Autodesk Fusion 360 part; units mm, degrees
note: some values were not read from the file. Set by a fixed rule: which face or edge a step refers to.
(part 2 of 5)
sketch "Sketch1 (5)" plane through (0, -26.65, 0) normal (0, -1, 0) x (1, 0, 0) in component "Servo_Mounting_Plate_1"
  line L0 (92.5, -27.97) -> (92.5, -18.97)
  line L1 (92.5, -18.97) -> (112.5, -18.97)
  line L2 (112.5, -18.97) -> (112.5, -27.97)
  line L3 (112.5, -27.97) -> (92.5, -27.97)
  circle A0 centre (11.5, -70.07) radius 1
  circle A1 centre (11.5, -4.1) radius 1
  circle A2 centre (11.5, -29.93) radius 1
  line L4 (92.5, -81.36) -> (92.5, -72.36)
  line L5 (92.5, -72.36) -> (112.5, -72.36)
  line L6 (112.5, -72.36) -> (112.5, -81.36)
  line L7 (112.5, -81.36) -> (92.5, -81.36)
  circle A3 centre (89.585, -23.47) radius 1
  circle A4 centre (115.415, -76.86) radius 1
  line L8 (16, -72.97) -> (16, -93)
  line L9 (16, -93) -> (7, -93)
  line L10 (7, -93) -> (7, -72.97)
  line L11 (7, -72.97) -> (16, -72.97)
  line L12 (16, -7) -> (16, -27.03)
  line L13 (16, -27.03) -> (7, -27.03)
  line L14 (7, -27.03) -> (7, -7)
  line L15 (7, -7) -> (16, -7)
  circle A5 centre (11.5, -95.9) radius 1
  circle A6 centre (89.585, -76.86) radius 1
  circle A7 centre (115.415, -23.47) radius 1
  line L16 (127.5, -73.5) -> (124.5, -73.5)
  line L17 (124.5, -73.5) -> (124.5, -68.5)
  line L18 (124.5, -68.5) -> (127.5, -68.5)
  line L19 (127.5, -68.5) -> (127.5, -73.5)
  line L20 (183.5, -73.5) -> (180.5, -73.5)
  line L21 (180.5, -73.5) -> (180.5, -68.5)
  line L22 (180.5, -68.5) -> (183.5, -68.5)
  line L23 (183.5, -68.5) -> (183.5, -73.5)
  line L24 (127.5, -31.5) -> (124.5, -31.5)
  line L25 (124.5, -31.5) -> (124.5, -26.5)
  line L26 (124.5, -26.5) -> (127.5, -26.5)
  line L27 (127.5, -26.5) -> (127.5, -31.5)
  line L28 (183.5, -31.5) -> (180.5, -31.5)
  line L29 (180.5, -31.5) -> (180.5, -26.5)
  line L30 (180.5, -26.5) -> (183.5, -26.5)
  line L31 (183.5, -26.5) -> (183.5, -31.5)
  arc A8 (157, -3) -> (154, 0) centre (154, -3) ccw
  line L32 (154, 0) -> (3, 0)
  arc A9 (3, 0) -> (0, -3) centre (3, -3) ccw
  line L33 (0, -3) -> (0, -97)
  arc A10 (0, -97) -> (3, -100) centre (3, -97) ccw
  line L34 (3, -100) -> (154, -100)
  arc A11 (154, -100) -> (157, -97) centre (154, -97) ccw
  line L35 (157, -97) -> (157, -94)
  arc A12 (160, -91) -> (157, -94) centre (160, -94) ccw
  line L36 (160, -91) -> (181.27, -91)
  arc A13 (181.27, -91) -> (184.27, -88) centre (181.27, -88) ccw
  line L37 (184.27, -88) -> (184.27, -12)
  arc A14 (184.27, -12) -> (181.27, -9) centre (181.27, -12) ccw
  line L38 (181.27, -9) -> (160, -9)
  arc A15 (157, -6) -> (160, -9) centre (160, -6) ccw
  line L39 (157, -6) -> (157, -3)
  line L40 (36.83, -3.81) -> (36.83, -13.97)
  line L41 (36.83, -13.97) -> (19.05, -13.97)
  line L42 (19.05, -13.97) -> (19.05, -3.81)
  line L43 (19.05, -3.81) -> (36.83, -3.81)
  line L44 (36.83, -96.52) -> (19.05, -96.52)
  line L45 (19.05, -96.52) -> (19.05, -86.36)
  line L46 (19.05, -86.36) -> (36.83, -86.36)
  line L47 (36.83, -86.36) -> (36.83, -96.52)
  line L48 (114.3, -3.81) -> (130.81, -3.81)
  line L49 (130.81, -3.81) -> (130.81, -13.97)
  line L50 (130.81, -13.97) -> (114.3, -13.97)
  line L51 (114.3, -13.97) -> (114.3, -3.81)
  line L52 (114.3, -96.52) -> (114.3, -86.36)
  line L53 (114.3, -86.36) -> (130.81, -86.36)
  line L54 (130.81, -86.36) -> (130.81, -96.52)
  line L55 (130.81, -96.52) -> (114.3, -96.52)
  circle A16 centre (115.415, -76.86) radius 1
  circle A17 centre (89.585, -76.86) radius 1
  line L56 (92.5, -76.86) -> (112.5, -76.86) construction
  line L57 (102.5, -72.36) -> (102.5, -81.36) construction
  line L58 (117.5, -86.25) -> (87.5, -86.25)
  line L59 (87.5, -86.25) -> (87.5, -67.47)
  line L60 (87.5, -67.47) -> (117.5, -67.47)
  line L61 (117.5, -67.47) -> (117.5, -86.25)
  line L62 (117.5, -86.25) -> (87.5, -67.47) construction
  line L63 (87.5, -86.25) -> (117.5, -67.47) construction
  line L64 (104.5, -72.36) -> (104.5, -81.36)
  line L65 (104.5, -72.36) -> (92.5, -72.36)
  line L66 (92.5, -72.36) -> (92.5, -81.36)
  line L67 (92.5, -81.36) -> (104.5, -81.36)
  point P0 (102.5, -76.86)
  dimension "d167" = 30
  dimension "d168" = 12
  constraint midpoint L4 L56.start
  constraint midpoint L6 L56.end
  constraint midpoint L5 L57.start
  constraint midpoint L7 L57.end
  constraint horizontal L58
  constraint perpendicular L58 L59
  constraint parallel L58 L60
  constraint parallel L59 L61
  constraint coincident L62 P0
  constraint coincident L63 P0
  constraint midpoint L57 P0
  constraint coincident L5 L64.start
  constraint coincident L7 L64.end
  constraint perpendicular L7 L64
  constraint coincident L4.end L5.start
  constraint coincident L4.start L7.end
  measures "d167" distance of L59.end L60.end
  measures "d168" distance of L4 L64
extrude "Extrude1''''''" add sketch "Sketch1 (5)" along normal blind 5.45 separate body contours L5 L6 L7 L64 | A4 A16 | A6 A17 | L58 L59 L60 L61 makes body 11 in component "Servo_Mounting_Plate_1"
sketch "Sketch2 (5)" plane through (0, -32.1, 0) normal (0, -1, 0) x (1, 0, 0) in component "Servo_Mounting_Plate_1"
  line L0 (92.5, -72.36) -> (104.5, -72.36)
  line L1 (104.5, -72.36) -> (104.5, -81.36)
  line L2 (104.5, -81.36) -> (92.5, -81.36)
  line L3 (92.5, -81.36) -> (92.5, -72.36)
  line L4 (117.5, -67.47) -> (87.5, -67.47)
  line L5 (87.5, -67.47) -> (87.5, -86.25)
  line L6 (87.5, -86.25) -> (117.5, -86.25)
  line L7 (117.5, -86.25) -> (117.5, -67.47)
  line L8 (92.5, -76.86) -> (96.3, -76.86) construction
  circle A0 centre (96.3, -76.86) radius 8.2
  circle A1 centre (96.3, -76.86) radius 10.2
  dimension "d171" = 3.8
  dimension "d172" = 2
  constraint midpoint L3 L8.start
  constraint perpendicular L3 L8
  constraint coincident L8.end A0.centre
  constraint tangent L1 A0
  measures "d171" distance of L8.start L8.end
extrude "Extrude2''''" cut sketch "Sketch2 (5)" against normal blind 2 contours L4 L5 L6 A1 bodies 11 in component "Servo_Mounting_Plate_1"
sketch "Sketch3 (3)" plane through (0, -26.65, 0) normal (0, 1, 0) x (-1, 0, 0) in component "Servo_Mounting_Plate_1"
  line L0 (-104.5, -72.36) -> (-92.5, -72.36)
  line L1 (-92.5, -72.36) -> (-92.5, -81.36)
  line L2 (-92.5, -81.36) -> (-104.5, -81.36)
  line L3 (-104.5, -81.36) -> (-104.5, -72.36)
  line L4 (-87.5, -67.47) -> (-117.5, -67.47)
  line L5 (-117.5, -67.47) -> (-117.5, -86.25)
  line L6 (-117.5, -86.25) -> (-87.5, -86.25)
  line L7 (-87.5, -86.25) -> (-87.5, -67.47)
  circle A0 centre (-90, -84) radius 0.95
  circle A1 centre (-90, -69.72) radius 0.95
  circle A2 centre (-114, -84) radius 0.95
  circle A3 centre (-114, -69.72) radius 0.95
  dimension "d175" = 2.25
  dimension "d176" = 2.25
  dimension "d177" = 2.25
  dimension "d178" = 2.25
  dimension "d314" = 1.9
  dimension "d315" = 24
  dimension "d316" = 1.9
  dimension "d317" = 1.9
  dimension "d318" = 1.9
  measures "d175" distance of L6 A0.centre
  measures "d176" distance of L4 A1.centre
  measures "d177" distance of L6 A2.centre
  measures "d178" distance of L4 A3.centre
  measures "d314" diameter of A0
  measures "d315" distance of A0.centre A2.centre
  measures "d316" diameter of A2
  measures "d317" diameter of A3
  measures "d318" diameter of A1
extrude "Extrude3''" add sketch "Sketch3 (3)" along normal blind 1 contours A0 | A1 | A2 | A3 bodies 11 in component "Servo_Mounting_Plate_1"
sketch "Sketch18" plane through (0, -26.65, 0) normal (0, -1, 0) x (1, 0, 0) in component "Chassis"
  line L0 (92.5, -27.97) -> (92.5, -18.97)
  line L1 (92.5, -18.97) -> (112.5, -18.97)
  line L2 (112.5, -18.97) -> (112.5, -27.97)
  line L3 (112.5, -27.97) -> (92.5, -27.97)
  circle A0 centre (11.5, -70.07) radius 1
  circle A1 centre (11.5, -4.1) radius 1
  circle A2 centre (11.5, -29.93) radius 1
  line L4 (92.5, -81.36) -> (92.5, -72.36)
  line L5 (92.5, -72.36) -> (112.5, -72.36)
  line L6 (112.5, -72.36) -> (112.5, -81.36)
  line L7 (112.5, -81.36) -> (92.5, -81.36)
  circle A3 centre (89.585, -23.47) radius 1
  circle A4 centre (115.415, -76.86) radius 1
  line L8 (16, -72.97) -> (16, -93)
  line L9 (16, -93) -> (7, -93)
  line L10 (7, -93) -> (7, -72.97)
  line L11 (7, -72.97) -> (16, -72.97)
  line L12 (16, -7) -> (16, -27.03)
  line L13 (16, -27.03) -> (7, -27.03)
  line L14 (7, -27.03) -> (7, -7)
  line L15 (7, -7) -> (16, -7)
  circle A5 centre (11.5, -95.9) radius 1
  circle A6 centre (89.585, -76.86) radius 1
  circle A7 centre (115.415, -23.47) radius 1
  line L16 (127.5, -73.5) -> (124.5, -73.5)
  line L17 (124.5, -73.5) -> (124.5, -68.5)
  line L18 (124.5, -68.5) -> (127.5, -68.5)
  line L19 (127.5, -68.5) -> (127.5, -73.5)
  line L20 (183.5, -73.5) -> (180.5, -73.5)
  line L21 (180.5, -73.5) -> (180.5, -68.5)
  line L22 (180.5, -68.5) -> (183.5, -68.5)
  line L23 (183.5, -68.5) -> (183.5, -73.5)
  line L24 (127.5, -31.5) -> (124.5, -31.5)
  line L25 (124.5, -31.5) -> (124.5, -26.5)
  line L26 (124.5, -26.5) -> (127.5, -26.5)
  line L27 (127.5, -26.5) -> (127.5, -31.5)
  line L28 (183.5, -31.5) -> (180.5, -31.5)
  line L29 (180.5, -31.5) -> (180.5, -26.5)
  line L30 (180.5, -26.5) -> (183.5, -26.5)
  line L31 (183.5, -26.5) -> (183.5, -31.5)
  arc A8 (157, -3) -> (154, 0) centre (154, -3) ccw
  line L32 (154, 0) -> (3, 0)
  arc A9 (3, 0) -> (0, -3) centre (3, -3) ccw
  line L33 (0, -3) -> (0, -97)
  arc A10 (0, -97) -> (3, -100) centre (3, -97) ccw
  line L34 (3, -100) -> (154, -100)
  arc A11 (154, -100) -> (157, -97) centre (154, -97) ccw
  line L35 (157, -97) -> (157, -94)
  arc A12 (160, -91) -> (157, -94) centre (160, -94) ccw
  line L36 (160, -91) -> (181.27, -91)
  arc A13 (181.27, -91) -> (184.27, -88) centre (181.27, -88) ccw
  line L37 (184.27, -88) -> (184.27, -12)
  arc A14 (184.27, -12) -> (181.27, -9) centre (181.27, -12) ccw
  line L38 (181.27, -9) -> (160, -9)
  arc A15 (157, -6) -> (160, -9) centre (160, -6) ccw
  line L39 (157, -6) -> (157, -3)
  line L40 (36.83, -3.81) -> (36.83, -13.97)
  line L41 (36.83, -13.97) -> (19.05, -13.97)
  line L42 (19.05, -13.97) -> (19.05, -3.81)
  line L43 (19.05, -3.81) -> (36.83, -3.81)
  line L44 (36.83, -96.52) -> (19.05, -96.52)
  line L45 (19.05, -96.52) -> (19.05, -86.36)
  line L46 (19.05, -86.36) -> (36.83, -86.36)
  line L47 (36.83, -86.36) -> (36.83, -96.52)
  line L48 (114.3, -3.81) -> (130.81, -3.81)
  line L49 (130.81, -3.81) -> (130.81, -13.97)
  line L50 (130.81, -13.97) -> (114.3, -13.97)
  line L51 (114.3, -13.97) -> (114.3, -3.81)
  line L52 (114.3, -96.52) -> (114.3, -86.36)
  line L53 (114.3, -86.36) -> (130.81, -86.36)
  line L54 (130.81, -86.36) -> (130.81, -96.52)
  line L55 (130.81, -96.52) -> (114.3, -96.52)
  circle A16 centre (90, -69.72) radius 1.0625
  circle A17 centre (90, -84) radius 1.0625
  circle A18 centre (114, -69.72) radius 1.0625
  circle A19 centre (114, -84) radius 1.0625
  line L56 (184.27, -50) -> (65, -50) construction
  circle A20 centre (90, -30.28) radius 1.0625
  circle A21 centre (114, -30.28) radius 1.0625
  circle A22 centre (114, -16) radius 1.0625
  circle A23 centre (90, -16) radius 1.0625
  point P0 (90, -69.72)
  point P1 (90, -84)
  point P2 (114, -84)
  point P3 (114, -69.72)
  dimension "d181" = 2.125
  dimension "d182" = 2.125
  dimension "d183" = 2.125
  dimension "d184" = 2.125
  constraint coincident P0 A16.centre
  constraint coincident P1 A17.centre
  constraint coincident P3 A18.centre
  constraint coincident P2 A19.centre
  constraint midpoint L37 L56.start
  constraint perpendicular L37 L56
  constraint symmetric A16 L56 A20
  constraint symmetric A17 L56 A23
  constraint symmetric A18 L56 A21
  constraint symmetric A19 L56 A22
  measures "d181" diameter of A16
  measures "d182" diameter of A17
  measures "d183" diameter of A18
  measures "d184" diameter of A19
extrude "Extrude17" cut sketch "Sketch18" against normal blind 1 contours A16 | A17 | A18 | A19 bodies 4 in component "Chassis"
extrude "Extrude18" cut sketch "Sketch18" against normal blind 1 contours A20 | A21 | A22 | A23 bodies 4 in component "Chassis"
sketch "Sketch1 (6)" plane through (0, -30.1, 0) normal (0, -1, 0) x (1, 0, 0) in component "Back_Wheel_L"
  arc A0 (103.1549, -72.36) -> (103.1549, -81.36) centre (96.3, -76.86) ccw
  line L0 (103.1549, -72.36) -> (104.5, -72.36)
  line L1 (104.5, -72.36) -> (104.5, -81.36)
  line L2 (104.5, -81.36) -> (103.1549, -81.36)
  arc A1 (100.2833, -86.25) -> (100.2833, -67.47) centre (96.3, -76.86) ccw
  line L3 (100.2833, -67.47) -> (92.3167, -67.47)
  arc A2 (92.3167, -67.47) -> (87.5, -71.7025) centre (96.3, -76.86) ccw
  line L4 (87.5, -71.7025) -> (87.5, -82.0175)
  arc A3 (87.5, -82.0175) -> (92.3167, -86.25) centre (96.3, -76.86) ccw
  line L5 (92.3167, -86.25) -> (100.2833, -86.25)
  circle A4 centre (96.3, -76.86) radius 10
  circle A5 centre (96.3, -76.86) radius 8.75
  dimension "d189" = 20
  dimension "d190" = -1.25
  constraint concentric A0 A4
  measures "d189" diameter of A4
extrude "Extrude1'''''''" add sketch "Sketch1 (6)" along normal blind 5.18 separate body contours L0 L1 A5 | L1 L2 A5 | L5 A4 | L3 L4 L5 A4 | L3 A4 | L4 A4 makes body 12 in component "Back_Wheel_L"
sketch "Sketch2 (6)" plane through (0, -35.28, 0) normal (0, -1, 0) x (1, 0, 0) in component "Back_Wheel_L"
  circle A0 centre (96.3, -76.86) radius 8.75
  circle A1 centre (96.3, -76.86) radius 10
  circle A2 centre (96.3, -76.86) radius 12
  dimension "d193" = 24
  constraint concentric A0 A2
  measures "d193" diameter of A2
extrude "Extrude2'''''" add sketch "Sketch2 (6)" against normal blind 3.15 contours A2 bodies 12 in component "Back_Wheel_L"
sketch "Sketch3 (4)" plane through (0, -35.28, 0) normal (0, -1, 0) x (1, 0, 0) in component "Back_Wheel_L"
  circle A0 centre (96.3, -76.86) radius 12
  circle A1 centre (96.3, -76.86) radius 8.75
  circle A2 centre (96.3, -76.86) radius 12
  constraint concentric A0 A2
extrude "Extrude3'''" add sketch "Sketch3 (4)" along normal blind 1 contours A0 A2 | A1 bodies 12 in component "Back_Wheel_L"
sketch "Sketch4 (3)" plane through (0, -36.28, 0) normal (0, -1, 0) x (1, 0, 0) in component "Back_Wheel_L"
  circle A0 centre (96.3, -76.86) radius 12
  circle A1 centre (96.3, -76.86) radius 8.75
  circle A2 centre (96.3, -76.86) radius 12
  constraint concentric A1 A2
extrude "Extrude4''" add sketch "Sketch4 (3)" along normal blind 10 bodies 12 in component "Back_Wheel_L"
sketch "Sketch5 (3)" plane through (0, -46.28, 0) normal (0, -1, 0) x (1, 0, 0) in component "Back_Wheel_L"
  circle A0 centre (96.3, -76.86) radius 8.75
  circle A1 centre (96.3, -76.86) radius 12
  line L0 (106, -76.86) -> (106, -69.7953)
  line L1 (106, -76.86) -> (106, -83.9247)
  line L2 (106, -83.9247) -> (111, -83.9247)
  line L3 (111, -83.9247) -> (111, -69.7953)
  line L4 (111, -69.7953) -> (106, -69.7953)
  line L5 (106, -69.7953) -> (106, -83.9247)
  dimension "d200" = 5
  constraint coincident A1 L0.end
  constraint coincident A1 L1.end
  constraint horizontal L2
  constraint vertical L3
  constraint horizontal L4
  constraint vertical L5
  measures "d200" distance of L1.end L2.end
extrude "Extrude5''" add sketch "Sketch5 (3)" against normal blind 10 contours A1 L2 L3 L4 bodies 12 in component "Back_Wheel_L"
sketch "Sketch6 (2)" plane through (0, 0, -83.9247) normal (0, 0, -1) x (-1, 0, 0) in component "Back_Wheel_L"
  line L0 (-111, -46.28) -> (-106, -46.28)
  line L1 (-106, -46.28) -> (-106, -36.28)
  line L2 (-106, -36.28) -> (-111, -36.28)
  line L3 (-111, -36.28) -> (-111, -46.28)
  line L4 (-111, -36.28) -> (-135.7487, -61.0287)
  line L5 (-111, -36.28) -> (-76, -36.28) construction
  line L6 (-135.7487, -61.0287) -> (-111, -46.28) construction
  line L7 (-135.7487, -61.0287) -> (-135.7487, -76.0287)
  line L8 (-135.7487, -76.0287) -> (-120.7487, -76.0287)
  line L9 (-120.7487, -76.0287) -> (-120.7487, -61.0287)
  line L10 (-111, -46.28) -> (-120.7487, -61.0287)
  dimension "d203" = 135
  dimension "d204" = 35
  dimension "d205" = 15
  dimension "d206" = 15
  dimension "d207" = 15
  constraint horizontal L5
  constraint coincident L2.end L3.start
  constraint coincident L0.start L3.end
  constraint vertical L7
  constraint perpendicular L7 L8
  constraint perpendicular L8 L9
  measures "d203" angle of L4 L5
  measures "d204" distance of L2.end L4.end
  measures "d205" distance of L4.end L7.end
  measures "d206" distance of L7.end L8.end
  measures "d207" distance of L8.end L9.end
extrude "Extrude6''" add sketch "Sketch6 (2)" against normal blind 14.129 contours L3 L4 L7 L8 L9 L10 bodies 12 in component "Back_Wheel_L"
sketch "Sketch1 (7)" plane through (0, -30.1, 0) normal (0, -1, 0) x (1, 0, 0) in component "Back_Wheel_R"
  arc A0 (103.1549, -72.36) -> (103.1549, -81.36) centre (96.3, -76.86) ccw
  line L0 (103.1549, -72.36) -> (104.5, -72.36)
  line L1 (104.5, -72.36) -> (104.5, -81.36)
  line L2 (104.5, -81.36) -> (103.1549, -81.36)
  arc A1 (100.2833, -86.25) -> (100.2833, -67.47) centre (96.3, -76.86) ccw
  line L3 (100.2833, -67.47) -> (92.3167, -67.47)
  arc A2 (92.3167, -67.47) -> (87.5, -71.7025) centre (96.3, -76.86) ccw
  line L4 (87.5, -71.7025) -> (87.5, -82.0175)
  arc A3 (87.5, -82.0175) -> (92.3167, -86.25) centre (96.3, -76.86) ccw
  line L5 (92.3167, -86.25) -> (100.2833, -86.25)
  circle A4 centre (96.3, -76.86) radius 10
  circle A5 centre (96.3, -76.86) radius 8.75
  dimension "d189_1" = 20
  dimension "d190_1" = -1.25
  constraint concentric A0 A4
  measures "d189_1" diameter of A4
extrude "Extrude1''''''''" add sketch "Sketch1 (7)" along normal blind 5.18 separate body contours L0 L1 A5 | L1 L2 A5 | L5 A4 | L3 L4 L5 A4 | L3 A4 | L4 A4 makes body 13 in component "Back_Wheel_R"
sketch "Sketch2 (7)" plane through (0, -35.28, 0) normal (0, -1, 0) x (1, 0, 0) in component "Back_Wheel_R"
  circle A0 centre (96.3, -76.86) radius 8.75
  circle A1 centre (96.3, -76.86) radius 10
  circle A2 centre (96.3, -76.86) radius 12
  dimension "d193_1" = 24
  constraint concentric A0 A2
  measures "d193_1" diameter of A2
extrude "Extrude2''''''" add sketch "Sketch2 (7)" against normal blind 3.15 contours A2 bodies 13 in component "Back_Wheel_R"
sketch "Sketch3 (5)" plane through (0, -35.28, 0) normal (0, -1, 0) x (1, 0, 0) in component "Back_Wheel_R"
  circle A0 centre (96.3, -76.86) radius 12
  circle A1 centre (96.3, -76.86) radius 8.75
  circle A2 centre (96.3, -76.86) radius 12
  constraint concentric A0 A2
extrude "Extrude3''''" add sketch "Sketch3 (5)" along normal blind 1 contours A0 A2 | A1 bodies 13 in component "Back_Wheel_R"
sketch "Sketch4 (4)" plane through (0, -36.28, 0) normal (0, -1, 0) x (1, 0, 0) in component "Back_Wheel_R"
  circle A0 centre (96.3, -76.86) radius 12
  circle A1 centre (96.3, -76.86) radius 8.75
  circle A2 centre (96.3, -76.86) radius 12
  constraint concentric A1 A2
extrude "Extrude4'''" add sketch "Sketch4 (4)" along normal blind 10 bodies 13 in component "Back_Wheel_R"
sketch "Sketch5 (4)" plane through (0, -46.28, 0) normal (0, -1, 0) x (1, 0, 0) in component "Back_Wheel_R"
  circle A0 centre (96.3, -76.86) radius 8.75
  circle A1 centre (96.3, -76.86) radius 12
  line L0 (106, -76.86) -> (106, -69.7953)
  line L1 (106, -76.86) -> (106, -83.9247)
  line L2 (106, -83.9247) -> (111, -83.9247)
  line L3 (111, -83.9247) -> (111, -69.7953)
  line L4 (111, -69.7953) -> (106, -69.7953)
  line L5 (106, -69.7953) -> (106, -83.9247)
  dimension "d200_1" = 5
  constraint coincident A1 L0.end
  constraint coincident A1 L1.end
  constraint horizontal L2
  constraint vertical L3
  constraint horizontal L4
  constraint vertical L5
  measures "d200_1" distance of L1.end L2.end
extrude "Extrude5'''" add sketch "Sketch5 (4)" against normal blind 10 contours A1 L2 L3 L4 bodies 13 in component "Back_Wheel_R"
sketch "Sketch6 (3)" plane through (0, 0, -83.9247) normal (0, 0, -1) x (-1, 0, 0) in component "Back_Wheel_R"
  line L0 (-111, -46.28) -> (-106, -46.28)
  line L1 (-106, -46.28) -> (-106, -36.28)
  line L2 (-106, -36.28) -> (-111, -36.28)
  line L3 (-111, -36.28) -> (-111, -46.28)
  line L4 (-111, -36.28) -> (-76, -36.28) construction
  line L5 (-135.7487, -61.0287) -> (-111, -46.28) construction
  line L6 (-135.7487, -61.0287) -> (-135.7487, -76.0287)
  line L7 (-135.7487, -76.0287) -> (-120.7487, -76.0287)
  line L8 (-120.7487, -76.0287) -> (-120.7487, -61.0287)
  line L9 (-120.7487, -61.0287) -> (-111, -46.28)
  line L10 (-111, -36.28) -> (-135.7487, -61.0287)
  dimension "d205_1" = 15
  dimension "d206_1" = 15
  dimension "d207_1" = 15
  constraint horizontal L4
  constraint coincident L2.end L3.start
  constraint coincident L0.start L3.end
  constraint vertical L6
  constraint perpendicular L6 L7
  constraint perpendicular L7 L8
  measures "d205_1" distance of L5.start L6.end
  measures "d206_1" distance of L6.end L7.end
  measures "d207_1" distance of L7.end L8.end
extrude "Extrude6'''" add sketch "Sketch6 (3)" against normal blind 14.129 contours L3 L6 L7 L8 L9 L10 bodies 13 in component "Back_Wheel_R"
sketch "Sketch2 (8)" plane through (0, -26.65, 0) normal (0, -1, 0) x (1, 0, 0) in component "Front_L_Servo_Mounting_Plate"
  circle A0 centre (90, -16) radius 1.0625
  circle A1 centre (114, -16) radius 1.0625
  circle A2 centre (90, -30.28) radius 1.0625
  circle A3 centre (114, -30.28) radius 1.0625
  circle A4 centre (114, -69.72) radius 1.0625
  circle A5 centre (90, -84) radius 1.0625
  circle A6 centre (90, -69.72) radius 1.0625
  circle A7 centre (114, -84) radius 1.0625
  line L0 (92.5, -27.97) -> (92.5, -18.97)
  line L1 (92.5, -18.97) -> (112.5, -18.97)
  line L2 (112.5, -18.97) -> (112.5, -27.97)
  line L3 (112.5, -27.97) -> (92.5, -27.97)
  circle A8 centre (11.5, -70.07) radius 1
  circle A9 centre (11.5, -4.1) radius 1
  circle A10 centre (11.5, -29.93) radius 1
  line L4 (92.5, -81.36) -> (92.5, -72.36)
  line L5 (92.5, -72.36) -> (112.5, -72.36)
  line L6 (112.5, -72.36) -> (112.5, -81.36)
  line L7 (112.5, -81.36) -> (92.5, -81.36)
  circle A11 centre (89.585, -23.47) radius 1
  circle A12 centre (115.415, -76.86) radius 1
  line L8 (16, -72.97) -> (16, -93)
  line L9 (16, -93) -> (7, -93)
  line L10 (7, -93) -> (7, -72.97)
  line L11 (7, -72.97) -> (16, -72.97)
  line L12 (16, -7) -> (16, -27.03)
  line L13 (16, -27.03) -> (7, -27.03)
  line L14 (7, -27.03) -> (7, -7)
  line L15 (7, -7) -> (16, -7)
  circle A13 centre (11.5, -95.9) radius 1
  circle A14 centre (89.585, -76.86) radius 1
  circle A15 centre (115.415, -23.47) radius 1
  line L16 (127.5, -73.5) -> (124.5, -73.5)
  line L17 (124.5, -73.5) -> (124.5, -68.5)
  line L18 (124.5, -68.5) -> (127.5, -68.5)
  line L19 (127.5, -68.5) -> (127.5, -73.5)
  line L20 (183.5, -73.5) -> (180.5, -73.5)
  line L21 (180.5, -73.5) -> (180.5, -68.5)
  line L22 (180.5, -68.5) -> (183.5, -68.5)
  line L23 (183.5, -68.5) -> (183.5, -73.5)
  line L24 (127.5, -31.5) -> (124.5, -31.5)
  line L25 (124.5, -31.5) -> (124.5, -26.5)
  line L26 (124.5, -26.5) -> (127.5, -26.5)
  line L27 (127.5, -26.5) -> (127.5, -31.5)
  line L28 (183.5, -31.5) -> (180.5, -31.5)
  line L29 (180.5, -31.5) -> (180.5, -26.5)
  line L30 (180.5, -26.5) -> (183.5, -26.5)
  line L31 (183.5, -26.5) -> (183.5, -31.5)
  arc A16 (157, -3) -> (154, 0) centre (154, -3) ccw
  line L32 (154, 0) -> (3, 0)
  arc A17 (3, 0) -> (0, -3) centre (3, -3) ccw
  line L33 (0, -3) -> (0, -97)
  arc A18 (0, -97) -> (3, -100) centre (3, -97) ccw
  line L34 (3, -100) -> (154, -100)
  arc A19 (154, -100) -> (157, -97) centre (154, -97) ccw
  line L35 (157, -97) -> (157, -94)
  arc A20 (160, -91) -> (157, -94) centre (160, -94) ccw
  line L36 (160, -91) -> (181.27, -91)
  arc A21 (181.27, -91) -> (184.27, -88) centre (181.27, -88) ccw
  line L37 (184.27, -88) -> (184.27, -12)
  arc A22 (184.27, -12) -> (181.27, -9) centre (181.27, -12) ccw
  line L38 (181.27, -9) -> (160, -9)
  arc A23 (157, -6) -> (160, -9) centre (160, -6) ccw
  line L39 (157, -6) -> (157, -3)
  line L40 (36.83, -3.81) -> (36.83, -13.97)
  line L41 (36.83, -13.97) -> (19.05, -13.97)
  line L42 (19.05, -13.97) -> (19.05, -3.81)
  line L43 (19.05, -3.81) -> (36.83, -3.81)
  line L44 (36.83, -96.52) -> (19.05, -96.52)
  line L45 (19.05, -96.52) -> (19.05, -86.36)
  line L46 (19.05, -86.36) -> (36.83, -86.36)
  line L47 (36.83, -86.36) -> (36.83, -96.52)
  line L48 (114.3, -3.81) -> (130.81, -3.81)
  line L49 (130.81, -3.81) -> (130.81, -13.97)
  line L50 (130.81, -13.97) -> (114.3, -13.97)
  line L51 (114.3, -13.97) -> (114.3, -3.81)
  line L52 (114.3, -96.52) -> (114.3, -86.36)
  line L53 (114.3, -86.36) -> (130.81, -86.36)
  line L54 (130.81, -86.36) -> (130.81, -96.52)
  line L55 (130.81, -96.52) -> (114.3, -96.52)
  line L56 (19.05, -86.36) -> (19.05, -100)
  line L57 (19.05, -100) -> (3, -100)
  line L58 (0, -97) -> (0, -68.36)
  line L59 (0, -68.36) -> (25, -68.36)
  line L60 (25, -68.36) -> (25, -86.36)
  line L61 (19.05, -86.36) -> (25, -86.36)
  arc A24 (0, -97) -> (3, -100) centre (3, -97) ccw
  line L62 (7, -72.97) -> (7, -84.97) construction
  line L63 (7, -84.97) -> (16, -84.97)
  dimension "d237" = 25
  dimension "d238" = 18
  dimension "d239" = 3
  dimension "d240" = 12
  constraint coincident L45.end L46.start
  constraint coincident L34 L56.end
  constraint perpendicular L34 L56
  constraint coincident A18.end L34.start
  constraint coincident L33.end A18.start
  constraint coincident L33 L58.end
  constraint perpendicular L34 L58
  constraint perpendicular L58 L59
  constraint coincident L46 L60.end
  constraint perpendicular L46 L60
  constraint coincident L10.end L11.start
  constraint perpendicular L11 L62
  constraint coincident L8 L63.end
  constraint perpendicular L8 L63
  measures "d237" distance of L58.end L59.end
  measures "d238" distance of L59.end L60.end
  measures "d239" radius of A24
  measures "d240" distance of L10.end L62.end
extrude "Extrude1'''''''''" add sketch "Sketch2 (8)" along normal blind 5.45 separate body contours A8 | L8 L9 L10 L63 | A13 | L33 A18 L34 L45 L46 L56 L57 L58 L59 L60 L61 A24 makes body 14 in component "Front_L_Servo_Mounting_Plate"
sketch "Sketch1 (8)" plane through (0, -32.1, 0) normal (0, -1, 0) x (1, 0, 0) in component "Front_L_Servo_Mounting_Plate"
  line L0 (7, -84.97) -> (7, -72.97)
  line L1 (7, -72.97) -> (16, -72.97)
  line L2 (16, -72.97) -> (16, -84.97)
  line L3 (16, -84.97) -> (7, -84.97)
  line L4 (0, -68.36) -> (0, -97)
  arc A0 (0, -97) -> (3, -100) centre (3, -97) ccw
  line L5 (3, -100) -> (19.05, -100)
  line L6 (19.05, -100) -> (19.05, -86.36)
  line L7 (19.05, -86.36) -> (25, -86.36)
  line L8 (25, -86.36) -> (25, -68.36)
  line L9 (25, -68.36) -> (0, -68.36)
  line L10 (11.5, -72.97) -> (11.5, -76.77) construction
  circle A1 centre (11.5, -76.77) radius 8.2
  circle A2 centre (11.5, -76.77) radius 10.2
  dimension "d243" = 3.8
  dimension "d244" = 2
  constraint midpoint L1 L10.start
  constraint perpendicular L1 L10
  constraint coincident L10.end A1.centre
  constraint tangent L3 A1
  measures "d243" distance of L10.start L10.end
extrude "Extrude2'''''''" cut sketch "Sketch1 (8)" against normal blind 2 contours L9 A2 picked at (13.8393, -85.5315) bodies 14 in component "Front_L_Servo_Mounting_Plate"
sketch "Sketch2 (9)" plane through (0, -26.65, 0) normal (0, 1, 0) x (-1, 0, 0) in component "Front_L_Servo_Mounting_Plate"
  line L0 (-7, -72.97) -> (-7, -84.97)
  line L1 (-7, -84.97) -> (-16, -84.97)
  line L2 (-16, -84.97) -> (-16, -72.97)
  line L3 (-16, -72.97) -> (-7, -72.97)
  line L4 (0, -97) -> (0, -68.36)
  line L5 (0, -68.36) -> (-25, -68.36)
  line L6 (-25, -68.36) -> (-25, -86.36)
  line L7 (-25, -86.36) -> (-19.05, -86.36)
  line L8 (-19.05, -86.36) -> (-19.05, -100)
  line L9 (-19.05, -100) -> (-3, -100)
  arc A0 (-3, -100) -> (0, -97) centre (-3, -97) ccw
  circle A1 centre (-3, -97) radius 0.95
  circle A2 centre (-22, -71) radius 0.95
  circle A3 centre (-3, -71) radius 0.95
  dimension "d247" = 1.9
  dimension "d249" = 1.9
  dimension "d250" = 1.9
  constraint concentric A0 A1
  measures "d247" diameter of A1
  measures "d249" diameter of A2
  measures "d250" diameter of A3
extrude "Extrude3'''''" add sketch "Sketch2 (9)" along normal blind 1 contours A1 | A2 | A3 bodies 14 in component "Front_L_Servo_Mounting_Plate"
sketch "Sketch19" plane through (0, -26.65, 0) normal (0, -1, 0) x (1, 0, 0) in component "Chassis"
  circle A0 centre (90, -16) radius 1.0625
  circle A1 centre (114, -16) radius 1.0625
  circle A2 centre (90, -30.28) radius 1.0625
  circle A3 centre (114, -30.28) radius 1.0625
  circle A4 centre (114, -69.72) radius 1.0625
  circle A5 centre (90, -84) radius 1.0625
  circle A6 centre (90, -69.72) radius 1.0625
  circle A7 centre (114, -84) radius 1.0625
  line L0 (92.5, -27.97) -> (92.5, -18.97)
  line L1 (92.5, -18.97) -> (112.5, -18.97)
  line L2 (112.5, -18.97) -> (112.5, -27.97)
  line L3 (112.5, -27.97) -> (92.5, -27.97)
  circle A8 centre (11.5, -70.07) radius 1
  circle A9 centre (11.5, -4.1) radius 1
  circle A10 centre (11.5, -29.93) radius 1
  line L4 (92.5, -81.36) -> (92.5, -72.36)
  line L5 (92.5, -72.36) -> (112.5, -72.36)
  line L6 (112.5, -72.36) -> (112.5, -81.36)
  line L7 (112.5, -81.36) -> (92.5, -81.36)
  circle A11 centre (89.585, -23.47) radius 1
  circle A12 centre (115.415, -76.86) radius 1
  line L8 (16, -72.97) -> (16, -93)
  line L9 (16, -93) -> (7, -93)
  line L10 (7, -93) -> (7, -72.97)
  line L11 (7, -72.97) -> (16, -72.97)
  line L12 (16, -7) -> (16, -27.03)
  line L13 (16, -27.03) -> (7, -27.03)
  line L14 (7, -27.03) -> (7, -7)
  line L15 (7, -7) -> (16, -7)
  circle A13 centre (11.5, -95.9) radius 1
  circle A14 centre (89.585, -76.86) radius 1
  circle A15 centre (115.415, -23.47) radius 1
  line L16 (127.5, -73.5) -> (124.5, -73.5)
  line L17 (124.5, -73.5) -> (124.5, -68.5)
  line L18 (124.5, -68.5) -> (127.5, -68.5)
  line L19 (127.5, -68.5) -> (127.5, -73.5)
  line L20 (183.5, -73.5) -> (180.5, -73.5)
  line L21 (180.5, -73.5) -> (180.5, -68.5)
  line L22 (180.5, -68.5) -> (183.5, -68.5)
  line L23 (183.5, -68.5) -> (183.5, -73.5)
  line L24 (127.5, -31.5) -> (124.5, -31.5)
  line L25 (124.5, -31.5) -> (124.5, -26.5)
  line L26 (124.5, -26.5) -> (127.5, -26.5)
  line L27 (127.5, -26.5) -> (127.5, -31.5)
  line L28 (183.5, -31.5) -> (180.5, -31.5)
  line L29 (180.5, -31.5) -> (180.5, -26.5)
  line L30 (180.5, -26.5) -> (183.5, -26.5)
  line L31 (183.5, -26.5) -> (183.5, -31.5)
  arc A16 (157, -3) -> (154, 0) centre (154, -3) ccw
  line L32 (154, 0) -> (3, 0)
  arc A17 (3, 0) -> (0, -3) centre (3, -3) ccw
  line L33 (0, -3) -> (0, -97)
  arc A18 (0, -97) -> (3, -100) centre (3, -97) ccw
  line L34 (3, -100) -> (154, -100)
  arc A19 (154, -100) -> (157, -97) centre (154, -97) ccw
  line L35 (157, -97) -> (157, -94)
  arc A20 (160, -91) -> (157, -94) centre (160, -94) ccw
  line L36 (160, -91) -> (181.27, -91)
  arc A21 (181.27, -91) -> (184.27, -88) centre (181.27, -88) ccw
  line L37 (184.27, -88) -> (184.27, -12)
  arc A22 (184.27, -12) -> (181.27, -9) centre (181.27, -12) ccw
  line L38 (181.27, -9) -> (160, -9)
  arc A23 (157, -6) -> (160, -9) centre (160, -6) ccw
  line L39 (157, -6) -> (157, -3)
  line L40 (36.83, -3.81) -> (36.83, -13.97)
  line L41 (36.83, -13.97) -> (19.05, -13.97)
  line L42 (19.05, -13.97) -> (19.05, -3.81)
  line L43 (19.05, -3.81) -> (36.83, -3.81)
  line L44 (36.83, -96.52) -> (19.05, -96.52)
  line L45 (19.05, -96.52) -> (19.05, -86.36)
  line L46 (19.05, -86.36) -> (36.83, -86.36)
  line L47 (36.83, -86.36) -> (36.83, -96.52)
  line L48 (114.3, -3.81) -> (130.81, -3.81)
  line L49 (130.81, -3.81) -> (130.81, -13.97)
  line L50 (130.81, -13.97) -> (114.3, -13.97)
  line L51 (114.3, -13.97) -> (114.3, -3.81)
  line L52 (114.3, -96.52) -> (114.3, -86.36)
  line L53 (114.3, -86.36) -> (130.81, -86.36)
  line L54 (130.81, -86.36) -> (130.81, -96.52)
  line L55 (130.81, -96.52) -> (114.3, -96.52)
  circle A24 centre (3, -97) radius 0.95 construction
  circle A25 centre (3, -71) radius 1 construction
  circle A26 centre (22, -71) radius 0.95 construction
  circle A27 centre (3, -97) radius 0.95 construction
  circle A28 centre (22, -71) radius 0.95 construction
  circle A29 centre (3, -71) radius 0.95 construction
  circle A30 centre (3, -71) radius 1.0625
  circle A31 centre (22, -71) radius 1.0625
  circle A32 centre (3, -97) radius 1.0625
  line L56 (0, -50) -> (31, -50) construction
  circle A33 centre (3, -29) radius 1.0625
  circle A34 centre (22, -29) radius 1.0625
  circle A35 centre (3, -3) radius 1.0625
  circle A36 centre (22, -71) radius 0.95
  circle A37 centre (3, -97) radius 0.95
  circle A38 centre (3, -71) radius 0.95
  point P0 (3, -97)
  point P1 (16, -97)
  point P2 (22, -71)
  point P3 (3, -71)
  point P4 (3, -97)
  point P5 (-1.5792, -95.1832)
  dimension "d253" = 2.125
  dimension "d254" = 2.125
  dimension "d255" = 2.125
  constraint coincident P3 A25.centre
  constraint concentric A26 A31
  constraint coincident P4 P0
  constraint midpoint L33 L56.start
  constraint perpendicular L33 L56
  constraint symmetric A30 L56 A33
  constraint symmetric A31 L56 A34
  constraint symmetric A32 L56 A35
  measures "d253" diameter of A30
  measures "d254" diameter of A31
  measures "d255" diameter of A32
extrude "Extrude20" cut sketch "Sketch19" against normal blind 1 contours A33 | A34 | A35 bodies 4 in component "Chassis"
extrude "Extrude19" cut sketch "Sketch19" against normal blind 1 contours A30 | A31 | A32 | A36 | A37 | A38 bodies 4 in component "Chassis"
sketch "Sketch7 (2)" plane through (0, 0, -30.4247) normal (0, 0, -1) x (-1, 0, 0)
  line L0 (-111, -46.28) -> (-106, -46.28)
  line L1 (-106, -46.28) -> (-106, -36.28)
  line L2 (-106, -36.28) -> (-111, -36.28)
  line L3 (-111, -36.28) -> (-135.7487, -61.0287)
  line L4 (-135.7487, -61.0287) -> (-135.7487, -76.0287)
  line L5 (-135.7487, -76.0287) -> (-120.7487, -76.0287)
  line L6 (-120.7487, -76.0287) -> (-120.7487, -61.0287)
  line L7 (-120.7487, -61.0287) -> (-111, -46.28)
  line L8 (-122.1487, -73.6287) -> (-134.3487, -73.6287)
  line L9 (-134.3487, -73.6287) -> (-134.3487, -63.4287)
  line L10 (-134.3487, -63.4287) -> (-122.1487, -63.4287)
  line L11 (-122.1487, -63.4287) -> (-122.1487, -73.6287)
  line L12 (-122.1487, -73.6287) -> (-134.3487, -63.4287) construction
  line L13 (-134.3487, -73.6287) -> (-122.1487, -63.4287) construction
  point P0 (-128.2487, -68.5287)
  dimension "d261" = 12.2
  dimension "d262" = 10.2
  constraint horizontal L8
  constraint perpendicular L8 L9
  constraint parallel L8 L10
  constraint parallel L9 L11
  constraint coincident L12 P0
  constraint coincident L13 P0
  measures "d261" distance of L9.end L10.end
  measures "d262" distance of L8.end L9.end
extrude "Extrude15'" cut sketch "Sketch7 (2)" against normal blind 12.97 contours L8 L9 L10 L11 sketch seen with x (1, 0, 0) y (0, 1, 0) z (0, 0, 1) at (0, 0, -53.5) bodies 13 in component "Back_Wheel_R"
sketch "Sketch4 (5)" plane through (0, 0, -30.4247) normal (0, 0, -1) x (-1, 0, 0)
sketch "Sketch14 (2)" plane through (0, 0, -70.9547) normal (0, 0, -1) x (-1, 0, 0) in component "Back_Wheel_R"
  line L0 (-122.1487, -63.4287) -> (-134.3487, -63.4287)
  line L1 (-134.3487, -63.4287) -> (-134.3487, -73.6287)
  line L2 (-134.3487, -73.6287) -> (-122.1487, -73.6287)
  line L3 (-122.1487, -73.6287) -> (-122.1487, -63.4287)
  circle A0 centre (-128.2487, -68.5287) radius 2
  line L4 (-128.2487, -68.5287) -> (-132.8207, -68.5287) construction
  line L5 (-128.2487, -68.5287) -> (-123.6767, -68.5287) construction
  circle A1 centre (-132.8207, -68.5287) radius 0.75
  circle A2 centre (-123.6767, -68.5287) radius 0.75
  dimension "d265" = 4
  dimension "d266" = 4.572
  dimension "d267" = 4.572
  dimension "d268" = 1.5
  dimension "d269" = 1.5
  constraint coincident A0.centre L4.start
  constraint perpendicular L1 L4
  constraint perpendicular L1 L5
  constraint coincident L4.end A1.centre
  constraint coincident L5.end A2.centre
  measures "d265" diameter of A0
  measures "d266" distance of A0.centre L4.end
  measures "d267" distance of A0.centre L5.end
  measures "d268" diameter of A1
  measures "d269" diameter of A2
extrude "Extrude16'" cut sketch "Sketch14 (2)" against normal blind 1.159 contours A0 | A1 | A2 bodies 13 in component "Back_Wheel_R"
sketch "Sketch15 (2)" plane through (55.9602, 36.989, 0) normal (-0.83423, -0.551416, 0) x (0, 0, 1) in component "Back_Wheel_R"
  line L0 (-83.9247, -99.8154) -> (-83.9247, -117.4948)
  line L1 (-83.9247, -117.4948) -> (-69.7957, -117.4948)
  line L2 (-69.7957, -117.4948) -> (-69.7957, -99.8154)
  line L3 (-69.7957, -99.8154) -> (-83.9247, -99.8154)
  line L4 (-82, -102) -> (-71.7204, -102)
  line L5 (-71.7204, -102) -> (-71.7204, -115.3102)
  line L6 (-71.7204, -115.3102) -> (-82, -115.3102)
  line L7 (-82, -115.3102) -> (-82, -102)
  line L8 (-82, -102) -> (-71.7204, -115.3102) construction
  line L9 (-71.7204, -102) -> (-82, -115.3102) construction
  point P0 (-76.8602, -108.6551)
  constraint horizontal L4
  constraint perpendicular L4 L5
  constraint parallel L4 L6
  constraint parallel L5 L7
  constraint coincident L8 P0
  constraint coincident L9 P0
extrude "Extrude17'" cut sketch "Sketch15 (2)" against normal blind 16 contours L4 L5 L6 L7 bodies 13 in component "Back_Wheel_R"
sketch "Sketch13 (2)" plane through (0, 0, -69.7957) normal (0, 0, 1) x (1, 0, 0) in component "Back_Wheel_L"
  line L0 (135.7487, -61.0287) -> (111, -36.28)
  line L1 (111, -36.28) -> (111, -46.28)
  line L2 (111, -46.28) -> (120.7487, -61.0287)
  line L3 (120.7487, -61.0287) -> (120.7487, -76.0287)
  line L4 (120.7487, -76.0287) -> (135.7487, -76.0287)
  line L5 (135.7487, -76.0287) -> (135.7487, -61.0287)
  line L6 (134.3487, -73.6287) -> (122.1487, -73.6287)
  line L7 (122.1487, -73.6287) -> (122.1487, -63.4287)
  line L8 (122.1487, -63.4287) -> (134.3487, -63.4287)
  line L9 (134.3487, -63.4287) -> (134.3487, -73.6287)
  line L10 (134.3487, -73.6287) -> (122.1487, -63.4287) construction
  line L11 (122.1487, -73.6287) -> (134.3487, -63.4287) construction
  point P0 (128.2487, -68.5287)
  dimension "d274" = 12.2
  dimension "d275" = 10.2
  constraint horizontal L6
  constraint perpendicular L6 L7
  constraint parallel L6 L8
  constraint parallel L7 L9
  constraint coincident L10 P0
  constraint coincident L11 P0
  measures "d274" distance of L7.end L8.end
  measures "d275" distance of L6.end L7.end
extrude "Extrude13'" cut sketch "Sketch13 (2)" against normal blind 12.97 contours L6 L7 L8 L9 bodies 12 in component "Back_Wheel_L"
sketch "Sketch14 (3)" plane through (0, 0, -82.7657) normal (0, 0, 1) x (1, 0, 0) in component "Back_Wheel_L"
  line L0 (134.3487, -63.4287) -> (122.1487, -63.4287)
  line L1 (122.1487, -63.4287) -> (122.1487, -73.6287)
  line L2 (122.1487, -73.6287) -> (134.3487, -73.6287)
  line L3 (134.3487, -73.6287) -> (134.3487, -63.4287)
  circle A0 centre (128.2487, -68.5287) radius 2
  line L4 (128.2487, -68.5287) -> (123.6767, -68.5287) construction
  line L5 (128.2487, -68.5287) -> (132.8207, -68.5287) construction
  circle A1 centre (123.6767, -68.5287) radius 0.75
  circle A2 centre (132.8207, -68.5287) radius 0.75
  dimension "d278" = 4
  dimension "d279" = 4.572
  dimension "d280" = 4.572
  dimension "d281" = 1.5
  dimension "d282" = 1.5
  constraint coincident A0.centre L4.start
  constraint perpendicular L1 L4
  constraint parallel L4 L5
  constraint coincident L4.end A1.centre
  constraint coincident L5.end A2.centre
  measures "d278" diameter of A0
  measures "d279" distance of A0.centre L4.end
  measures "d280" distance of A0.centre L5.end
  measures "d281" diameter of A1
  measures "d282" diameter of A2
extrude "Extrude14'" cut sketch "Sketch14 (3)" against normal blind 1.159 contours A0 | A1 | A2 bodies 12 in component "Back_Wheel_L"
sketch "Sketch15 (3)" plane through (55.9602, 36.989, 0) normal (-0.83423, -0.551416, 0) x (0, 0, 1) in component "Back_Wheel_L"
  line L0 (-83.9247, -99.8154) -> (-83.9247, -117.4948)
  line L1 (-83.9247, -117.4948) -> (-69.7957, -117.4948)
  line L2 (-69.7957, -117.4948) -> (-69.7957, -99.8154)
  line L3 (-69.7957, -99.8154) -> (-83.9247, -99.8154)
  line L4 (-82.0002, -115.3101) -> (-71.7202, -115.3101)
  line L5 (-71.7202, -115.3101) -> (-71.7202, -102.0001)
  line L6 (-71.7202, -102.0001) -> (-82.0002, -102.0001)
  line L7 (-82.0002, -102.0001) -> (-82.0002, -115.3101)
  line L8 (-82.0002, -115.3101) -> (-71.7202, -102.0001) construction
  line L9 (-71.7202, -115.3101) -> (-82.0002, -102.0001) construction
  point P0 (-76.8602, -108.6551)
  dimension "d285" = 10.28
  dimension "d286" = 13.31
  constraint horizontal L4
  constraint perpendicular L4 L5
  constraint parallel L4 L6
  constraint parallel L5 L7
  constraint coincident L8 P0
  constraint coincident L9 P0
  measures "d285" distance of L5.end L6.end
  measures "d286" distance of L4.end L5.end
extrude "Extrude15''" cut sketch "Sketch15 (3)" against normal blind 15 contours L4 L5 L6 L7 bodies 12 in component "Back_Wheel_L"
sketch "Sketch16 (2)" plane through (0, -35.28, 0) normal (0, 1, 0) x (-1, 0, 0) in component "Back_Wheel_L"
  circle A0 centre (-96.3, -76.86) radius 8.75
  circle A1 centre (-96.3, -76.86) radius 2.25
  dimension "d289" = 4.5
  constraint concentric A0 A1
  measures "d289" diameter of A1
extrude "Extrude16''" cut sketch "Sketch16 (2)" against normal blind 1 contours A1 bodies 12 in component "Back_Wheel_L"
sketch "Sketch17 (2)" plane through (0, -35.28, 0) normal (0, 1, 0) x (-1, 0, 0) in component "Back_Wheel_L"
  circle A0 centre (-96.3, -76.86) radius 2.25
  circle A1 centre (-96.3, -76.86) radius 8.75
  line L0 (-96.3, -68.11) -> (-96.3, -85.61) construction
  line L1 (-105.05, -76.86) -> (-87.55, -76.86) construction
  line L2 (-104.9098, -78.42) -> (-97.86, -78.42)
  line L3 (-94.74, -78.42) -> (-87.6902, -78.42)
  line L4 (-97.86, -68.2502) -> (-97.86, -75.3)
  line L5 (-97.86, -78.42) -> (-97.86, -85.4698)
  line L6 (-94.74, -68.2502) -> (-94.74, -75.3)
  line L7 (-94.74, -78.42) -> (-94.74, -85.4698)
  line L8 (-104.9098, -75.3) -> (-97.86, -75.3)
  line L9 (-94.74, -75.3) -> (-87.6902, -75.3)
  constraint coincident A1 L0.start
  constraint coincident A1 L0.end
  constraint coincident A1 L1.start
  constraint coincident A1 L1.end
  constraint perpendicular L0 L1
  constraint parallel L1 L2
  constraint coincident L3.start L6
  constraint collinear L2 L3
  constraint coincident L2.end L4
  constraint parallel L0 L4
  constraint collinear L4 L5
  constraint parallel L0 L6
  constraint coincident L6.end L8
  constraint collinear L6 L7
  constraint parallel L1 L8
  constraint collinear L8 L9
  constraint coincident A1 L2.start
  constraint coincident A1 L5.end
  constraint coincident A1 L7.end
  constraint coincident A1 L3.end
  constraint coincident A1 L9.end
  constraint coincident A1 L6.start
  constraint coincident A1 L4.start
  constraint coincident A1 L8.start
extrude "Extrude17''" add sketch "Sketch17 (2)" along normal blind 1 contours A0 L6 L9 | A0 A1 L6 L9 | A0 A1 L3 L7 | A0 L3 L7 | A0 L4 L8 | A0 A1 L4 L8 | A0 A1 L2 L5 | A0 L2 L5 bodies 12 in component "Back_Wheel_L"
sketch "Sketch16 (3)" plane through (0, -35.28, 0) normal (0, 1, 0) x (-1, 0, 0) in component "Back_Wheel_R"
  circle A0 centre (-96.3, -76.86) radius 8.75
  circle A1 centre (-96.3, -76.86) radius 2.25
  dimension "d298" = 4.5
  constraint concentric A0 A1
  measures "d298" diameter of A1
extrude "Extrude18'" cut sketch "Sketch16 (3)" against normal blind 1 contours A1 bodies 13 in component "Back_Wheel_R"
sketch "Sketch17 (3)" plane through (0, -35.28, 0) normal (0, 1, 0) x (-1, 0, 0) in component "Back_Wheel_R"
  circle A0 centre (-96.3, -76.86) radius 2.25
  circle A1 centre (-96.3, -76.86) radius 8.75
  line L0 (-105.05, -76.86) -> (-87.55, -76.86) construction
  line L1 (-96.3, -68.11) -> (-96.3, -85.61) construction
  line L2 (-94.74, -68.2502) -> (-94.74, -75.3)
  line L3 (-94.74, -78.42) -> (-94.74, -85.4698)
  line L4 (-104.9098, -78.42) -> (-97.86, -78.42)
  line L5 (-94.74, -78.42) -> (-87.6902, -78.42)
  line L6 (-104.9098, -75.3) -> (-97.86, -75.3)
  line L7 (-94.74, -75.3) -> (-87.6902, -75.3)
  line L8 (-97.86, -68.2502) -> (-97.86, -75.3)
  line L9 (-97.86, -78.42) -> (-97.86, -85.4698)
  constraint coincident A1 L0.start
  constraint coincident A1 L0.end
  constraint horizontal L0
  constraint coincident A1 L1.start
  constraint coincident A1 L1.end
  constraint perpendicular L0 L1
  constraint parallel L1 L2
  constraint coincident L3.start L4
  constraint collinear L2 L3
  constraint parallel L0 L4
  constraint collinear L4 L5
  constraint coincident L4.end L8
  constraint parallel L0 L6
  constraint collinear L6 L7
  constraint parallel L1 L8
  constraint collinear L8 L9
  constraint coincident A1 L5.end
  constraint coincident A1 L7.end
  constraint coincident A1 L2.start
  constraint coincident A1 L8.start
  constraint coincident A1 L6.start
  constraint coincident A1 L4.start
  constraint coincident A1 L3.end
  constraint coincident A1 L9.end
extrude "Extrude19'" add sketch "Sketch17 (3)" along normal blind 1 contours A0 L2 L7 | A0 A1 L2 L7 | A0 A1 L3 L5 | A0 L3 L5 | A0 L6 L8 | A0 A1 L6 L8 | A0 A1 L4 L9 | A0 L4 L9 bodies 13 in component "Back_Wheel_R"
fillet "Fillet2''" radius 2 4 edges at (94.74, -34.78, -75.3) (97.86, -34.78, -75.3) (94.74, -34.78, -78.42) (97.86, -34.78, -78.42) on bodies 12 in component "Back_Wheel_L"
fillet "Fillet2'''" radius 2 4 edges at (97.86, -34.78, -78.42) (97.86, -34.78, -75.3) (94.74, -34.78, -78.42) (94.74, -34.78, -75.3) on bodies 13 in component "Back_Wheel_R"
sketch "Sketch4 (6)" plane through (0, -26.65, 0) normal (0, 1, 0) x (-1, 0, 0) in component "Servo_Mounting_Plate_1"
  circle A0 centre (-90, -84) radius 0.95
  circle A1 centre (-114, -84) radius 0.95
  circle A2 centre (-90, -69.72) radius 0.95
  circle A3 centre (-114, -69.72) radius 0.95
  line L0 (-104.5, -72.36) -> (-92.5, -72.36)
  line L1 (-92.5, -72.36) -> (-92.5, -81.36)
  line L2 (-92.5, -81.36) -> (-104.5, -81.36)
  line L3 (-104.5, -81.36) -> (-104.5, -72.36)
  line L4 (-87.5, -67.47) -> (-117.5, -67.47)
  line L5 (-117.5, -67.47) -> (-117.5, -86.25)
  line L6 (-117.5, -86.25) -> (-87.5, -86.25)
  line L7 (-87.5, -86.25) -> (-87.5, -67.47)
  line L8 (-117.5, -70.946) -> (-87.5, -70.946)
  line L9 (-87.5, -82.774) -> (-117.5, -82.774)
  line L10 (-117.5, -82.774) -> (-117.5, -70.946)
  line L11 (-117.5, -70.946) -> (-87.5, -80.2839) construction
  line L12 (-87.5, -73.4361) -> (-117.5, -82.774) construction
  line L13 (-87.5, -82.774) -> (-87.5, -70.946)
  point P0 (-98.5, -76.86)
  dimension "d309" = 3.4761
  dimension "d310" = 3.4761
  dimension "d311" = 11.828
  constraint horizontal L8
  constraint parallel L8 L9
  constraint coincident L5 L8.start
  constraint coincident L11 P0
  constraint coincident L12 P0
  constraint coincident L7 L9.start
  constraint coincident L7 L8.end
  constraint coincident L7 L11.end
  constraint coincident L7 L12.start
  measures "d309" distance of L6 L9
  measures "d310" distance of L4 L8
  measures "d311" distance of L8.start L9.end
extrude "Extrude4''''" cut sketch "Sketch4 (6)" against normal blind 1.5 contours L5 L7 L8 L9 L10 L13 bodies 11 in component "Servo_Mounting_Plate_1"
sketch "Sketch3 (1)" plane through (0, -26.65, 0) normal (0, 1, 0) x (-1, 0, 0) in component "Front_L_Servo_Mounting_Plate"
  circle A0 centre (-22, -71) radius 0.95
  circle A1 centre (-3, -71) radius 0.95
  circle A2 centre (-3, -97) radius 0.95
  line L0 (-7, -72.97) -> (-7, -84.97)
  line L1 (-7, -84.97) -> (-16, -84.97)
  line L2 (-16, -84.97) -> (-16, -72.97)
  line L3 (-16, -72.97) -> (-7, -72.97)
  line L4 (0, -97) -> (0, -68.36)
  line L5 (0, -68.36) -> (-25, -68.36)
  line L6 (-25, -68.36) -> (-25, -86.36)
  line L7 (-25, -86.36) -> (-19.05, -86.36)
  line L8 (-19.05, -86.36) -> (-19.05, -100)
  line L9 (-19.05, -100) -> (-3, -100)
  arc A3 (-3, -100) -> (0, -97) centre (-3, -97) ccw
  line L10 (-17.5498, -100) -> (-5.4502, -100)
  line L11 (-5.4502, -100) -> (-5.4502, -68.36)
  line L12 (-17.5498, -68.36) -> (-17.5498, -100)
  line L13 (-17.5498, -100) -> (-8.4478, -68.36) construction
  line L14 (-5.4502, -100) -> (-14.5522, -68.36) construction
  line L15 (-5.4502, -68.36) -> (-17.5498, -68.36)
  point P0 (-11.5, -78.97)
  dimension "d319" = 7.4502
  dimension "d320" = 5.4502
  constraint horizontal L10
  constraint perpendicular L10 L11
  constraint parallel L11 L12
  constraint coincident L9 L10.start
  constraint coincident L13 P0
  constraint coincident L14 P0
  constraint coincident L5 L12.start
  constraint coincident L5 L11.end
  constraint coincident L5 L13.end
  constraint coincident L5 L14.end
  measures "d319" distance of L6 L12
  measures "d320" distance of L4 L11
extrude "Extrude4'''''" cut sketch "Sketch3 (1)" against normal blind 1.5 contours L5 L9 L10 L11 L12 L15 bodies 14 in component "Front_L_Servo_Mounting_Plate"